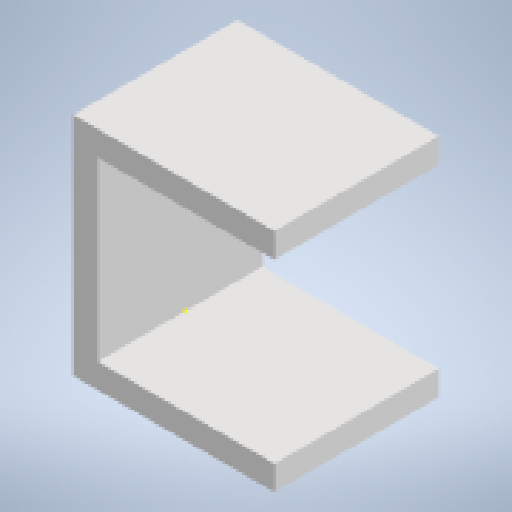
# Autodesk Inventor part: Держатель
Saved by Autodesk Inventor 2023 (Build 270158000, 158)
## iProperties
Created: 2023-04-09
Part Number: Держатель
Material: Типовые
Document SubType Name: Modeling
Designer: deryu
Density: 1 g/cm^3
Appearance: По умолчанию
Author: deryu
Autodesk Inventor part; units mm, degrees
ref_plane "YZ Plane" through (0, 0, 0) normal (1, 0, 0) x (0, 1, 0)
ref_plane "XZ Plane" through (0, 0, 0) normal (0, 1, 0) x (-1, 0, 0)
sketch "Эскиз1" plane through (0, 0, 0) normal (0, 0, 1) x (1, 0, 0)
  line L0 (21.5, 21.5) -> (21.5, -21.5)
  line L1 (21.5, -21.5) -> (-21.5, -21.5)
  line L2 (-21.5, -21.5) -> (-21.5, 21.5)
  line L3 (-21.5, 21.5) -> (21.5, 21.5)
  line L4 (21.5, 21.5) -> (-21.5, -21.5) construction
  line L5 (21.5, -21.5) -> (-21.5, 21.5) construction
  circle A0 centre (15.5, -15.5) radius 1.55 projected
  circle A1 centre (-15.5, -15.5) radius 1.55 projected
  circle A2 centre (-15.5, 15.5) radius 1.55 projected
  circle A3 centre (15.5, 15.5) radius 1.55 projected
  line L6 (21.5, -21.5) -> (21.5, -27.5)
  line L7 (21.5, -27.5) -> (-27.5, -27.5)
  line L8 (-27.5, -27.5) -> (-27.5, 27.5)
  line L9 (-27.5, 27.5) -> (21.5, 27.5)
  line L10 (21.5, 27.5) -> (21.5, 21.5)
  point P0 (0, 0)
  dimension "d0" = 43
  dimension "d1" = 43
  dimension "d2" = 6
  dimension "d3" = 49
  dimension "d4" = 55
  constraints: 22 end point, 5 perpendicular, 2 midpoint, 2 parallel, 2 vertical, 1 point on line
  measures "d0" distance of L0.start L0.end
  measures "d1" distance of L0.end L1.end
  measures "d2" distance of L0.end L6.end
  measures "d3" distance of L6.end L7.end
  measures "d4" distance of L7.end L8.end
ref_plane "РабПлоскость1" through (-20.5, -20.5, -40) normal (0, 0, -1) x (0, 1, 0)
extrude "Выдавливание1" add sketch "Эскиз1" against normal up to surface (40 mm away) contours L3 L2 L1 L6 L7 L8 L9 L10
sketch "Эскиз3" plane through (0, 0, 0) normal (0, 0, 1) x (1, 0, 0)
  circle A0 centre (15.5, -15.5) radius 1.55 projected
  circle A1 centre (-15.5, -15.5) radius 1.55 projected
  circle A2 centre (-15.5, 15.5) radius 1.55 projected
  circle A3 centre (15.5, 15.5) radius 1.55 projected
  line L0 (-27.5, -27.5) -> (21.5, -27.5) projected
  line L1 (21.5, -21.5) -> (21.5, -27.5) projected
  line L2 (21.5, 21.5) -> (21.5, -21.5) projected
  line L3 (21.5, 27.5) -> (21.5, 21.5) projected
  line L4 (21.5, 27.5) -> (-27.5, 27.5) projected
  line L5 (-27.5, 27.5) -> (-27.5, -27.5) projected
  point P0 (0, 0)
extrude "Выдавливание2" add sketch "Эскиз3" along normal blind 3
